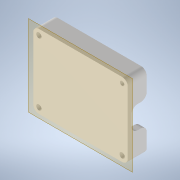
# Autodesk Inventor part: ESP32ParasiteMicroscope_bottom_v0
Saved by Autodesk Inventor 2022 (Build 260153000, 153)
## iProperties
Created: 2022-03-17
Part Number: ESP32ParasiteMicroscope_bottom_v0
Material: Generic
Document SubType Name: Modeling
Designer: Prakash Lab
Density: 1 g/cm^3
Appearance: Default
Author: Prakash Lab
Autodesk Inventor part; units mm, degrees
ref_plane "YZ Plane" through (0, 0, 0) normal (1, 0, 0) x (0, 1, 0)
ref_plane "XZ Plane" through (0, 0, 0) normal (0, 1, 0) x (-1, 0, 0)
ref_plane "Work Plane1" through (0, 0, 10) normal (0, 0, 1) x (1, 0, 0)
sketch "Sketch1" plane through (0, 0, 10) normal (0, 0, 1) x (1, 0, 0)
  arc A0 (-19.968, 15.1761) -> (-17.968, 13.1761) centre (-17.968, 15.1761) ccw projected
  line L0 (-17.968, 13.1761) -> (12.6451, 13.1761) projected
  line L1 (12.6451, 13.1761) -> (12.6451, 10.1761) projected
  line L2 (12.6451, 10.1761) -> (-8.2819, 10.1761) projected
  arc A1 (-8.2819, 10.1761) -> (-10.2819, 8.1761) centre (-8.2819, 8.1761) ccw projected
  line L3 (-10.2819, 8.1761) -> (-10.2819, 6.2345) projected
  arc A2 (-12.2819, 4.2345) -> (-10.2819, 6.2345) centre (-12.2819, 6.2345) ccw projected
  line L4 (-12.2819, 4.2345) -> (-17.968, 4.2345) projected
  arc A3 (-17.968, 4.2345) -> (-19.968, 2.2345) centre (-17.968, 2.2345) ccw projected
  line L5 (-19.968, 2.2345) -> (-19.968, -16.4874) projected
  arc A4 (-19.968, -16.4874) -> (-16.968, -19.4874) centre (-16.968, -16.4874) ccw projected
  line L6 (-16.968, -19.4874) -> (27.032, -19.4874) projected
  arc A5 (27.032, -19.4874) -> (30.032, -16.4874) centre (27.032, -16.4874) ccw projected
  line L7 (30.032, -16.4874) -> (30.032, 16.4874) projected
  arc A6 (30.032, 16.4874) -> (27.032, 19.4874) centre (27.032, 16.4874) ccw projected
  line L8 (27.032, 19.4874) -> (-16.968, 19.4874) projected
  arc A7 (-16.968, 19.4874) -> (-19.968, 16.4874) centre (-16.968, 16.4874) ccw projected
  line L9 (-19.968, 16.4874) -> (-19.968, 15.1761) projected
  line L10 (-15.2819, -12.7969) -> (-15.2819, -9.7969) projected
  line L11 (-15.2819, -9.7969) -> (12.6451, -9.7969) projected
  line L12 (12.6451, -9.7969) -> (12.6451, -12.7969) projected
  line L13 (12.6451, -12.7969) -> (-15.2819, -12.7969) projected
  circle A8 centre (-16.968, 16.4874) radius 1.4 projected
  circle A9 centre (27.032, -16.4874) radius 1.4 projected
  circle A10 centre (-16.968, -16.4874) radius 1.4 projected
  circle A11 centre (27.032, 16.4874) radius 1.15 projected
  line L14 (-19.968, 2.2345) -> (-19.968, 15.8318)
  point P0 (0, 0)
  constraints: 2 end point, 1 midpoint
extrude "Extrusion1" add sketch "Sketch1" against normal blind 2 contours L9 A7 L8 A6 L7 A5 L6 A4 L5 A3 L4 A2 L3 A1 L2 L1 L0 A0 | A0 L0 L1 L2 A1 L3 A2 L4 A3 L14 | L10 L11 L12 L13
sketch "Sketch2" plane through (0, 0, 8) normal (0, 0, -1) x (-1, 0, 0)
  arc A0 (16.968, -19.4874) -> (19.968, -16.4874) centre (16.968, -16.4874) ccw projected
  line L0 (19.968, -16.4874) -> (19.968, 16.4874) projected
  arc A1 (19.968, 16.4874) -> (16.968, 19.4874) centre (16.968, 16.4874) ccw projected
  line L1 (16.968, 19.4874) -> (-27.032, 19.4874) projected
  arc A2 (-27.032, 19.4874) -> (-30.032, 16.4874) centre (-27.032, 16.4874) ccw projected
  line L2 (-30.032, 16.4874) -> (-30.032, -16.4874) projected
  arc A3 (-30.032, -16.4874) -> (-27.032, -19.4874) centre (-27.032, -16.4874) ccw projected
  line L3 (-27.032, -19.4874) -> (16.968, -19.4874) projected
  circle A4 centre (-27.032, 16.4874) radius 1.15 projected
  circle A5 centre (16.968, -16.4874) radius 1.4 projected
  circle A6 centre (-27.032, -16.4874) radius 1.4 projected
  circle A7 centre (16.968, 16.4874) radius 1.4 projected
  line L4 (-24.732, 16.1874) -> (14.668, 16.1874)
  line L5 (16.668, 14.1874) -> (16.668, -14.1874)
  line L6 (14.668, -16.1874) -> (-24.732, -16.1874)
  line L7 (-26.732, -14.1874) -> (-26.732, 14.1874)
  line L8 (-24.0716, 16.1874) -> (-11.323, 16.1874) projected
  arc A8 (-24.732, 16.1874) -> (-26.732, 14.1874) centre (-24.732, 14.1874) ccw
  arc A9 (16.668, 14.1874) -> (14.668, 16.1874) centre (14.668, 14.1874) ccw
  arc A10 (14.668, -16.1874) -> (16.668, -14.1874) centre (14.668, -14.1874) ccw
  arc A11 (-26.732, -14.1874) -> (-24.732, -16.1874) centre (-24.732, -14.1874) ccw
  line L9 (-30.032, 6) -> (-26.732, 6)
  line L10 (-30.032, -16.4874) -> (-30.032, 16.4874) projected
  line L11 (-30.032, -6) -> (-26.732, -6)
  point P0 (0, 0)
  point P1 (15.6957, 15.9032)
  point P2 (16.3837, 15.2152)
  point P3 (16.3837, -15.2152)
  point P4 (15.6957, -15.9032)
  point P5 (-25.7597, -15.9032)
  point P6 (-26.4477, -15.2152)
  dimension "d2" = 2
  dimension "d3" = 6
  dimension "d4" = 6
  constraints: 12 end point, 8 point on circle, 8 tangent, 5 point on line, 4 centre point, 3 equal radius, 1 horizontal, 1 perpendicular, 3 other
  measures "d2" radius of A8
  measures "d3" distance from line of L9 point (0, 0)
  measures "d4" distance from line of point (0, 0) L11
ref_plane "Work Plane2" through (-19.968, -19.4874, 0) normal (0, 0, 1) x (1, 0, 0)
extrude "Extrusion2" add sketch "Sketch2" along normal up to surface (8 mm away) contours L3 A3 L2 L11 L7 A11 A6 L6 A10 A5 L5 A9 A7 L4 A8 L9 A2 L1 A1 L0 A0
fillet "Fillet1" radius 3.175 4 edges at (28.382, 6, 8) (28.382, 6, 0) (28.382, -6, 8) (28.382, -6, 0)
body "Solid1"
